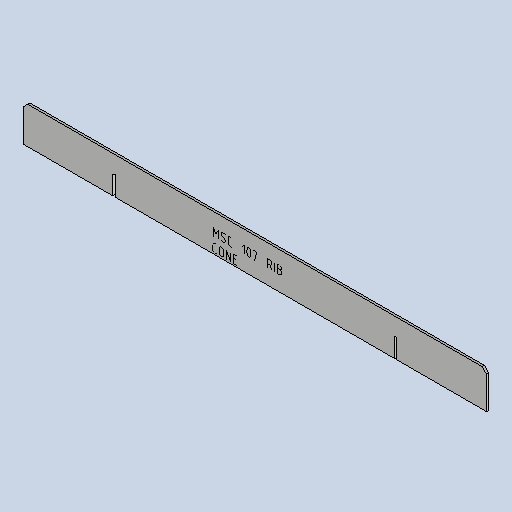
# Autodesk Inventor part: MSC 107 RIB CONE
Saved by Autodesk Inventor 2025 (Build 290162010, 162A)
## iProperties
Created: 2024-06-26
Part Number: MSC 107 RIB CONE
Material: Stainless Steel
Document SubType Name: Sheet Metal
Designer: pokla
Density: 8 g/cm^3
Sheet Metal Rule: AISI304 3mm Die 32
Appearance: Default
Stock Number: МОО 107 шпангоут конус
Mass: 751.267 g
Surface Area: 669.765 cm^2
Volume: 93.9084 cm^3
Flat Pattern Width: 5 cm
Flat Pattern Length: 63 cm
Flat Pattern Area: 315 cm^2
Sheet Metal Width: 50,000 mm
Sheet Metal Length: 630,000 mm
Sheet Metal Area: 31500,000 mm^2
Author: pokla
Autodesk Inventor part; units mm, degrees
ref_plane "YZ Plane" through (0, 0, 0) normal (1, 0, 0) x (0, 1, 0)
ref_plane "XZ Plane" through (0, 0, 0) normal (0, 1, 0) x (-1, 0, 0)
ref_plane "XY Plane" through (0, 0, 0) normal (0, 0, 1) x (1, 0, 0)
sketch "Sketch2" plane through (0, 0, 0) normal (0, 1, 0) x (-1, 0, 0)
  line L0 (375, 50) -> (-375, 50)
  line L1 (-375, 50) -> (-375, 0)
  line L2 (-375, 0) -> (375, 0)
  line L3 (375, 0) -> (375, 50)
  circle A0 centre (-375, 0) radius 22.5
  circle A1 centre (375, 0) radius 22.5
  point P0 (0, 0)
  point P1 (0, 0)
  point P2 (-375, 22.5)
  point P3 (-352.5, 0)
  point P4 (352.5, 0)
  point P5 (375, 22.5)
  dimension "d18" = 750
  dimension "d19" = 50
  dimension "d20" = 45
  measures "d18" distance of L2.end L1.end
  measures "d19" distance of L1.end L0.end
  measures "d20" diameter of A0
extrude "Plate2" add sketch "Sketch2" along normal blind 3 contours L3 A1 L2 A0 L1 L0 | L3 L2 A1 | A0 L2 L1 picked at (360.188, 1.6689) picked at (-360.9308, 4.923)
sketch "Sketch3" plane through (0, 3, 0) normal (0, 1, 0) x (1, 0, 0)
  line L0 (-191.55, 0) -> (-191.55, -50) construction
  line L1 (-375, -50) -> (375, -50) construction
  line L2 (-375, -50) -> (-375, 0) projected
  line L3 (-193.1, 0) -> (-190, 0)
  line L4 (-190, 0) -> (-190, -26)
  line L5 (-190, -26) -> (-193.1, -26)
  line L6 (-193.1, -26) -> (-193.1, 0)
  line L7 (-375, 0) -> (375, 0) projected
  line L8 (375, 0) -> (-375, 0) projected
  line L9 (191.55, 0) -> (191.55, -50) construction
  line L10 (190, -26) -> (193.1, -26)
  line L11 (193.1, -26) -> (193.1, 0)
  line L12 (193.1, 0) -> (190, 0)
  line L13 (190, 0) -> (190, -26)
  line L14 (0, 0) -> (0, -50) construction
  point P0 (0, 0)
  point P1 (0, 0)
  point P2 (190, 0)
  point P3 (193.1, 0)
  dimension "d24" = 26
  dimension "d44" = 3.1
  dimension "d45" = 380
  constraints: 22 end point, 4 midpoint, 4 parallel, 3 perpendicular, 3 point on line, 2 equal length, 2 horizontal, 1 vertical, 4 other
  measures "d24" distance of L3.end L4.end
  measures "d44" distance of L4.end L5.end
  measures "d45" distance between parallel lines of L13 L4
extrude "Extrusion1" cut sketch "Sketch3" against normal through all
sketch "Sketch4" plane through (0, 3, 0) normal (0, 1, 0) x (1, 0, 0)
  line L0 (-190, 0) -> (-190, -26) projected
  line L1 (-190, -26) -> (-193.1, -26) projected
  line L2 (-193.1, -26) -> (-193.1, 0) projected
  line L3 (-375, 0) -> (-193.1, 0) projected
  line L4 (-375, -50) -> (-375, 0) projected
  line L5 (375, -50) -> (-375, -50) projected
  line L6 (375, 0) -> (375, -50) projected
  line L7 (193.1, 0) -> (375, 0) projected
  line L8 (190, -26) -> (190, 0) projected
  line L9 (193.1, -26) -> (190, -26) projected
  line L10 (193.1, 0) -> (193.1, -26) projected
  line L11 (-190, 0) -> (190, 0) projected
  line L12 (-193.1, 0) -> (-375, 0) projected
  line L13 (-315, 0) -> (-315, -50)
  line L14 (315, 0) -> (315, -50)
  line L15 (-375, -50) -> (375, -50) projected
  point P0 (0, 0)
  dimension "d35" = 60
  dimension "d36" = 60
  constraints: 4 end point, 4 point on line, 1 parallel, 1 perpendicular
  measures "d35" distance between parallel lines of L4 L13
  measures "d36" distance between parallel lines of L6 L14
extrude "Extrusion2" cut sketch "Sketch4" against normal through all contours L13 L5 L4 L3 | L7 L6 L5 L14
sketch "Sketch5" plane through (0, 0, 0) normal (0, -1, 0) x (1, 0, 0)
  line L0 (-57.747, 1.3029) -> (-57.747, 31.8939) construction
  line L1 (-57.747, 31.8939) -> (64.2813, 31.8939) construction
  line L2 (64.2813, 31.8939) -> (64.2813, 1.3029) construction
  line L3 (64.2813, 1.3029) -> (-57.747, 1.3029) construction
  point P0 (0, 0)
  constraints: 2 other
mark "Mark1"
chamfer "Corner Chamfer1" distance 6 angle 45 2 edges at (-315, 1.5, 50) (315, 1.5, 50)
equation "\"d36\" = d35"
equation "\"d21\" = Thickness"
equation "\"BendReliefWidth\" = Thickness"
equation "\"BendReliefDepth\" = 0.5 * Thickness"
equation "\"CornerReliefSize\" = 4 * Thickness"
equation "\"MinimumRemnant\" = 2 * Thickness"
equation "\"TransitionRadius\" = BendRadius"
equation "\"JacobiRadiusSize\" = BendRadius"
equation "\"GapSize\" = Thickness"
equation "\"Thickness\" = 3"
equation "\"BendRadius\" = 5"
body "Solid2"
